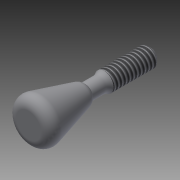
# Autodesk Inventor part: peg
Saved by Autodesk Inventor 2015 (Build 190159000, 159)
## iProperties
Created: 2015-04-06
Part Number: peg
Material: Generic
Document SubType Name: Modeling
Designer: WASHHSST
Density: 1 g/cm^3
Appearance: Default
Author: WASHHSST
Autodesk Inventor part; units mm, degrees
ref_plane "YZ Plane" through (0, 0, 0) normal (1, 0, 0) x (0, 1, 0)
ref_plane "XZ Plane" through (0, 0, 0) normal (0, 1, 0) x (-1, 0, 0)
ref_plane "XY Plane" through (0, 0, 0) normal (0, 0, 1) x (1, 0, 0)
sketch "Sketch1" plane through (0, 0, 0) normal (0, 0, 1) x (1, 0, 0)
  circle A0 centre (0, 0) radius 3.175
  dimension "d0" = 6.35
  constraints: 1 centre point, 1 coincident
  measures "d0" diameter of A0
extrude "Extrusion1" add sketch "Sketch1" along normal blind 15.875
thread "Thread1" size "1/4-20 UNC" class "2A" standard "ANSI Unified Screw Threads" full length
chamfer "Chamfer1" distance 1.27 angle 45 1 edges at (-3.175, 0, 0)
sketch "Sketch3" plane through (0, 0, 15.875) normal (0, 0, 1) x (1, 0, 0)
  circle A0 centre (0, 0) radius 2.54
  dimension "d11" = 5.08
  constraints: 1 centre point, 1 coincident
  measures "d11" diameter of A0
extrude "Extrusion3" add sketch "Sketch3" along normal blind 6.35
sketch "Sketch4" plane through (0, 0, 22.225) normal (0, 0, 1) x (1, 0, 0)
  circle A0 centre (0, 0) radius 3.175
  dimension "d14" = 6.35
  constraints: 1 centre point, 1 coincident
  measures "d14" diameter of A0
extrude "Extrusion4" add sketch "Sketch4" along normal blind 19.05 draft 15
fillet "Fillet2" radius 3.175 3 edges at (-8.2794, 0, 41.275) (-3.175, 0, 22.225) (-2.54, 0, 15.875)
body "Solid1"
